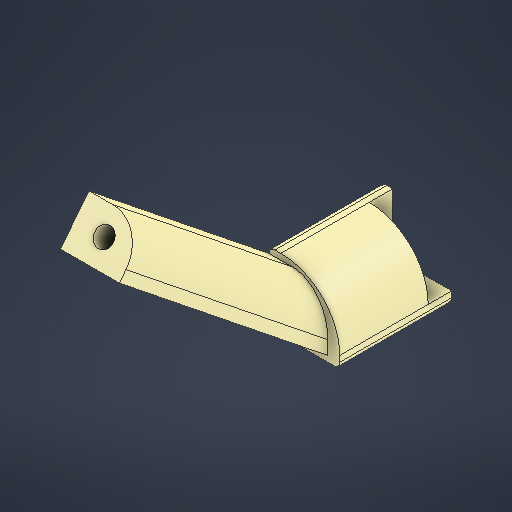
# Autodesk Inventor part: display_top_support_right
Saved by Autodesk Inventor 2026 (Build 300175050, 175E)
## iProperties
Created: 2025-06-09
Part Number: display_top_support_right
Material: Generic
Document SubType Name: Modeling
Designer: satom
Density: 1 g/cm^3
Appearance: Default
Author: satom
Autodesk Inventor part; units mm, degrees
ref_plane "YZ Plane" through (0, 0, 0) normal (1, 0, 0) x (0, 1, 0)
ref_plane "XZ Plane" through (0, 0, 0) normal (0, 1, 0) x (-1, 0, 0)
ref_plane "XY Plane" through (0, 0, 0) normal (0, 0, 1) x (1, 0, 0)
sketch "Sketch1" plane through (0, 0, 0) normal (0, 0, 1) x (1, 0, 0)
  line L0 (0, 0) -> (12.7, 0)
  line L1 (0, 0) -> (0, 12.7)
  arc A0 (12.7, 0) -> (0, 12.7) centre (0, 0) ccw
  circle A1 centre (5.08, 5.08) radius 3.1115
  dimension "d0" = 12.7
  dimension "d2" = 6.223
  dimension "d3" = 5.08
  dimension "d4" = 5.08
  constraints: 4 end point, 2 centre point, 2 point on circle, 1 coincident, 1 horizontal, 1 vertical
  measures "d0" distance of L0.start L1.end
  measures "d2" diameter of A1
  measures "d3" distance from line of L0 A1.centre
  measures "d4" distance from line of L1 A1.centre
extrude "Extrusion1" add sketch "Sketch1" along normal blind 3.81
sketch "Sketch2" plane through (0, 0, 0) normal (0, 0, -1) x (-1, 0, 0)
  arc A0 (0, 12.7) -> (-12.7, 0) centre (0, 0) ccw projected
  line L0 (0, 12.7) -> (0, 0) projected
  line L1 (0, 12.7) -> (0, 0)
  line L2 (0, 0) -> (-12.7, 0) projected
  line L3 (-12.7, 0) -> (0, 0)
  line L4 (0, 12.7) -> (1.27, 12.7)
  line L5 (-12.7, 0) -> (-12.7, -1.27)
  line L6 (-11.43, -2.54) -> (1.27, -2.54)
  line L7 (2.54, -1.27) -> (2.54, 11.43)
  arc A1 (2.54, 11.43) -> (1.27, 12.7) centre (1.27, 11.43) ccw
  arc A2 (1.27, -2.54) -> (2.54, -1.27) centre (1.27, -1.27) ccw
  arc A3 (-12.7, -1.27) -> (-11.43, -2.54) centre (-11.43, -1.27) ccw
  point P0 (2.54, 12.7)
  point P1 (-12.7, -2.54)
  dimension "d7" = 2.54
  dimension "d8" = 2.54
  dimension "d9" = 1.27
  constraints: 12 end point, 6 point on circle, 6 tangent, 4 point on line, 3 centre point, 3 perpendicular, 2 equal radius, 1 collinear, 1 horizontal, 1 parallel
  measures "d7" distance of L0.start point (2.54, 12.7)
  measures "d8" distance of L2.end point (-12.7, -2.54)
  measures "d9" radius of A1
extrude "Extrusion2" add sketch "Sketch2" along normal blind 5.08 and the other way blind 3.81 contours L4 A1 L7 A2 L6 A3 L5 L2 L0
sketch "Sketch3" plane through (0, 0, 3.81) normal (0, 0, 1) x (1, 0, 0)
  circle A0 centre (5.08, 5.08) radius 3.1115 projected
  circle A1 centre (5.08, 5.08) radius 1.2
  arc A2 (12.7, 0) -> (0, 12.7) centre (0, 0) ccw projected
  arc A3 (12.7, 0) -> (0, 12.7) centre (0, 0) ccw
  line L0 (-1.27, -2.54) -> (11.43, -2.54)
  line L1 (12.7, -1.27) -> (12.7, 0)
  line L2 (-2.54, -1.27) -> (-2.54, 11.43)
  line L3 (-1.27, 12.7) -> (0, 12.7)
  arc A4 (11.43, -2.54) -> (12.7, -1.27) centre (11.43, -1.27) ccw
  arc A5 (-2.54, -1.27) -> (-1.27, -2.54) centre (-1.27, -1.27) ccw
  arc A6 (-1.27, 12.7) -> (-2.54, 11.43) centre (-1.27, 11.43) ccw
  point P0 (-2.54, -2.54)
  point P1 (12.7, -2.54)
  point P2 (-2.54, 12.7)
  dimension "d14" = 2.4
  dimension "d15" = 15.24
  dimension "d16" = 15.24
  dimension "d17" = 1.27
  constraints: 8 end point, 8 point on circle, 8 tangent, 6 point on line, 5 centre point, 2 coincident, 2 equal radius, 2 perpendicular, 1 horizontal, 1 vertical
  measures "d14" diameter of A1
  measures "d15" distance of point (-2.54, -2.54) point (12.7, -2.54)
  measures "d16" distance of point (-2.54, -2.54) point (-2.54, 12.7)
  measures "d17" radius of A4
extrude "Extrusion3" add sketch "Sketch3" along normal blind 2.54 contours A0 | L1 A4 L0 A5 L2 A6 L3 A2
sketch "Sketch4" plane through (0, 0, 6.35) normal (0, 0, 1) x (1, 0, 0)
  line L0 (0, 0) -> (12.7, 0) projected
  line L1 (-1.27, 12.7) -> (0, 12.7) projected
  arc A0 (12.7, 0) -> (0, 12.7) centre (0, 0) ccw
  line L2 (0, 12.7) -> (-1.27, 12.7)
  line L3 (-2.54, 11.43) -> (-2.54, -1.27)
  line L4 (-1.27, -2.54) -> (11.43, -2.54)
  line L5 (12.7, -1.27) -> (12.7, 0)
  arc A1 (-1.27, 12.7) -> (-2.54, 11.43) centre (-1.27, 11.43) ccw
  arc A2 (-2.54, -1.27) -> (-1.27, -2.54) centre (-1.27, -1.27) ccw
  arc A3 (11.43, -2.54) -> (12.7, -1.27) centre (11.43, -1.27) ccw
  circle A4 centre (5.08, 5.08) radius 1.2 projected
  circle A5 centre (5.08, 5.08) radius 3.175
  point P0 (-2.54, 12.7)
  point P1 (-2.54, -2.54)
  point P2 (12.7, -2.54)
  dimension "d20" = 15.24
  dimension "d21" = 15.24
  dimension "d22" = 1.27
  dimension "d23" = 6.35
  constraints: 8 end point, 8 point on circle, 7 tangent, 6 point on line, 5 centre point, 3 perpendicular, 2 coincident, 2 equal radius, 1 horizontal
  measures "d20" distance of point (-2.54, -2.54) point (12.7, -2.54)
  measures "d21" distance of point (-2.54, 12.7) point (-2.54, -2.54)
  measures "d22" radius of A1
  measures "d23" diameter of A5
extrude "Extrusion4" add sketch "Sketch4" along normal blind 12.7 contours L1 A0 L5 A3 L4 A2 L3 A1
sketch "Sketch5" plane through (-2.54, -1.27, -5.08) normal (-1, 0, 0) x (0, 0, 1)
  line L0 (24.13, 0) -> (0, 0) projected
  line L1 (24.13, 0) -> (69.0907, 35.9945)
  line L2 (24.13, 12.7) -> (0, 12.7) projected
  line L3 (24.13, 12.7) -> (62.8946, 43.7341)
  line L4 (69.0907, 35.9945) -> (62.8946, 43.7341)
  line L5 (24.13, 12.7) -> (24.13, 13.97) projected
  line L6 (24.13, 12.7) -> (24.13, 0)
  point P0 (5.08, 1.27)
  dimension "d26" = 141.32
  dimension "d27" = 141.32
  dimension "d28" = 57.594
  constraints: 8 end point, 2 perpendicular
  measures "d26" angle of L0 L1
  measures "d27" angle of L2 L3
  measures "d28" distance of L0.start L1.end
extrude "Extrusion5" add sketch "Sketch5" against normal blind 12.7
sketch "Sketch6" plane through (0, 0, 19.05) normal (0, 0, 1) x (1, 0, 0)
  circle A0 centre (5.08, 5.08) radius 1.2 projected
  circle A1 centre (5.08, 5.08) radius 3.1115
  point P0 (0, 0)
  dimension "d31" = 6.223
  constraints: 1 centre point, 1 coincident
  measures "d31" diameter of A1
extrude "Extrusion6" cut sketch "Sketch6" along normal blind 12.7 contours A0 | A1
sketch "Sketch7" plane through (-2.54, 34.7245, 64.0107) normal (0, 0.6249702, 0.7806486) x (1, 0, 0)
  line L0 (8.0758, 9.9142) -> (12.7, 9.9142) construction
  line L1 (12.7, 0) -> (0, 0) construction
  line L2 (12.7, 9.9142) -> (0, 0) construction
  line L3 (0, 0) -> (0, 15.0805) construction
  line L4 (0, 9.9142) -> (12.7, 0) construction
  circle A0 centre (6.35, 4.9571) radius 2
  point P0 (2.54, 12.8971)
  dimension "d34" = 4
  constraints: 4 end point, 1 centre point, 1 midpoint, 1 point on line
  measures "d34" diameter of A0
extrude "Extrusion7" cut sketch "Sketch7" against normal blind 7
fillet "Fillet1" radius 7.62 1 edges at (10.16, 26.947, 38.4323)
equation "\"d34\" = m3_heat_set_insert"
equation "\"d35\" = m3_heat_set_depth"
equation "\"m3_heat_set_insert\" = 4"
equation "\"m3_clearance\" = 3.4"
equation "\"m3_heat_set_depth\" = 7"
equation "\"robot_diameter\" = 354"
equation "\"hardboard_thickness\" = 5"
body "Solid1"
